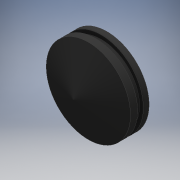
# Autodesk Inventor part: Plunger Rubber
Saved by Autodesk Inventor 2018 (Build 220112000, 112)
## iProperties
Created: 2019-11-16
Part Number: Plunger Rubber
Material: Generic
Document SubType Name: Modeling
Designer: ASUS
Density: 1 g/cm^3
Appearance: Rubber - Black
Author: ASUS
Autodesk Inventor part; units mm, degrees
ref_plane "YZ Plane" through (0, 0, 0) normal (1, 0, 0) x (0, 1, 0)
ref_plane "XZ Plane" through (0, 0, 0) normal (0, 1, 0) x (-1, 0, 0)
ref_plane "XY Plane" through (0, 0, 0) normal (0, 0, 1) x (1, 0, 0)
sketch "Sketch1" plane through (0, 0, 0) normal (0, 0, 1) x (1, 0, 0)
  line L0 (0.7333, 10.3377) -> (-10.2667, 10.3377)
  line L1 (-10.2667, 10.3377) -> (-10.2667, 8.8377)
  line L2 (-10.2667, 8.8377) -> (-9.2667, 8.8377)
  line L3 (-9.2667, 8.8377) -> (-9.2667, 7.3377)
  line L4 (-9.2667, 7.3377) -> (-10.2667, 7.3377)
  line L5 (-10.2667, 7.3377) -> (-10.2667, 5.4877)
  line L6 (-10.2667, 5.4877) -> (0.7333, 1.484)
  line L7 (0.7333, 1.484) -> (0.7333, 10.3377)
  point P0 (0, 0)
  dimension "d0" = 20
  dimension "d1" = 10
  dimension "d2" = 1.5
  dimension "d3" = 1.5
  dimension "d4" = 1.85
  dimension "d5" = 11
  constraints: 16 end point, 4 perpendicular, 2 point on line, 1 horizontal, 1 parallel
  measures "d0" angle of L6 L0
  measures "d1" distance between parallel lines of L7 L3
  measures "d2" distance of L0.end L1.end
  measures "d3" distance of L2.end L3.end
  measures "d4" distance of L4.end L5.end
  measures "d5" distance of L0.start L0.end
revolve "Revolution1" add sketch "Sketch1" angle 360 about axis through (0.7333, 1.484, 0) along (0, 1, 0)
sketch "Sketch2" plane through (0, 0, 0) normal (0, 0, 1) x (1, 0, 0)
  line L0 (11.7333, 5.4877) -> (-10.2667, 5.4877) projected
  line L1 (0.7333, 5.4877) -> (0.7333, 11.4877)
  line L2 (0.7333, 5.4877) -> (-6.7667, 5.4877)
  line L3 (-6.7667, 8.4877) -> (-5.2667, 8.4877)
  line L4 (-5.2667, 8.4877) -> (-5.2667, 11.4877)
  line L5 (-5.2667, 11.4877) -> (0.7333, 11.4877)
  line L6 (-6.7667, 8.4877) -> (-6.7667, 5.4877)
  point P0 (0, 0)
  dimension "d7" = 6
  dimension "d8" = 3
  dimension "d9" = 7.5
  dimension "d10" = 3
  dimension "d11" = 6
  constraints: 12 end point, 2 perpendicular, 2 vertical, 1 horizontal, 1 midpoint, 1 point on line
  measures "d7" distance of L1.start L1.end
  measures "d8" distance of L3.end L4.end
  measures "d9" distance of L2.end L1.start
  measures "d10" distance of L3.start L2.end
  measures "d11" distance of L4.end L1.end
revolve "Revolution2" cut sketch "Sketch2" angle 360 about axis through (0.7333, 5.4877, 0) along (0, 1, 0)
body "Solid1"
